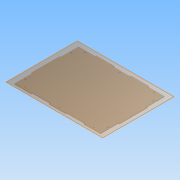
# Autodesk Inventor part: right part
Saved by Autodesk Inventor 2017 (Build 210142000, 142)
## iProperties
Part Number: right part
Material: Типовые
Document SubType Name: Modeling
Designer: Max
Mass: 338.04 g
Surface Area: 1748.93 cm^2
Volume: 338.04 cm^3
Density: 1 g/cm^3
Appearance: Поликарбонат — дымчатый
Author: Max
Autodesk Inventor part; units mm, degrees
ref_plane "YZ Plane" through (0, 0, 0) normal (1, 0, 0) x (0, 1, 0)
ref_plane "XZ Plane" through (0, 0, 0) normal (0, 1, 0) x (-1, 0, 0)
ref_plane "XY Plane" through (0, 0, 0) normal (0, 0, 1) x (1, 0, 0)
ref_plane "РабПлоскость1" through (0, 0, 0) normal (0, 0, 1) x (1, 0, 0)
sketch "Эскиз1" plane through (0, 0, 0) normal (0, 0, 1) x (1, 0, 0)
  line L0 (-1.5, 574) -> (-1.5, 579)
  line L1 (-1.5, 579) -> (-32.8, 579)
  line L2 (-32.8, 579) -> (-32.8, 583)
  line L3 (-32.8, 583) -> (-102.7, 583)
  line L4 (-102.7, 583) -> (-102.7, 579)
  line L5 (-102.7, 579) -> (-133.85, 579)
  line L6 (-133.85, 579) -> (-133.85, 574)
  line L7 (-133.85, 574) -> (-132.55, 574)
  line L8 (-132.55, 574) -> (-132.55, 571.55)
  line L9 (-132.55, 571.55) -> (-133.85, 571.55)
  line L10 (-133.85, 571.55) -> (-133.85, 570.5)
  line L11 (-133.85, 570.5) -> (-136.85, 570.5)
  line L12 (-136.85, 570.5) -> (-136.85, 571.55)
  line L13 (-136.85, 571.55) -> (-138.15, 571.55)
  line L14 (-138.15, 571.55) -> (-138.15, 574)
  line L15 (-138.15, 574) -> (-136.85, 574)
  line L16 (-136.85, 574) -> (-136.85, 579)
  line L17 (-136.85, 579) -> (-168, 579)
  line L18 (-168, 579) -> (-168, -179)
  line L19 (-168, -179) -> (168, -179)
  line L20 (168, -179) -> (168, 579)
  line L21 (168, 579) -> (136.85, 579)
  line L22 (136.85, 579) -> (136.85, 574)
  line L23 (136.85, 574) -> (138.15, 574)
  line L24 (138.15, 574) -> (138.15, 571.55)
  line L25 (138.15, 571.55) -> (136.85, 571.55)
  line L26 (136.85, 571.55) -> (136.85, 570.5)
  line L27 (136.85, 570.5) -> (133.85, 570.5)
  line L28 (133.85, 570.5) -> (133.85, 571.55)
  line L29 (133.85, 571.55) -> (132.55, 571.55)
  line L30 (132.55, 571.55) -> (132.55, 574)
  line L31 (132.55, 574) -> (133.85, 574)
  line L32 (133.85, 574) -> (133.85, 579)
  line L33 (133.85, 579) -> (102.7, 579)
  line L34 (102.7, 579) -> (102.7, 583)
  line L35 (102.7, 583) -> (32.8, 583)
  line L36 (32.8, 583) -> (32.8, 579)
  line L37 (32.8, 579) -> (1.5, 579)
  line L38 (1.5, 579) -> (1.5, 574)
  line L39 (1.5, 574) -> (2.8, 574)
  line L40 (2.8, 574) -> (2.8, 571.55)
  line L41 (2.8, 571.55) -> (1.5, 571.55)
  line L42 (1.5, 571.55) -> (1.5, 570.5)
  line L43 (1.5, 570.5) -> (-1.5, 570.5)
  line L44 (-1.5, 570.5) -> (-1.5, 571.55)
  line L45 (-1.5, 571.55) -> (-2.8, 571.55)
  line L46 (-2.8, 571.55) -> (-2.8, 574)
  line L47 (-2.8, 574) -> (-1.5, 574)
  circle A0 centre (138, 299) radius 4.75
  line L48 (-143, 100.6) -> (-143, 130)
  line L49 (-143, 130) -> (-121.6, 130)
  line L50 (-121.6, 130) -> (-121.6, 100.6)
  line L51 (-121.6, 100.6) -> (-143, 100.6)
  circle A1 centre (-156.5, 22) radius 2
  circle A2 centre (156.5, 50) radius 2
  circle A3 centre (156.5, -165) radius 2
  circle A4 centre (156.5, 132) radius 2
  circle A5 centre (-156.5, 132) radius 2
  circle A6 centre (-156.5, -165) radius 2
  circle A7 centre (158, 171) radius 5
  circle A8 centre (156, 144) radius 5
  circle A9 centre (-158, 171) radius 5
  circle A10 centre (-156, 144) radius 5
  line L52 (39.6112, -91.2079) -> (39.6112, -93.7719)
  line L53 (39.6112, -93.7719) -> (32.3927, -93.7719)
  line L54 (32.3927, -93.7719) -> (32.3927, -95.6776)
  line L55 (32.3927, -95.6776) -> (39.0914, -95.6776)
  line L56 (39.0914, -95.6776) -> (39.0914, -98.1261)
  line L57 (39.0914, -98.1261) -> (32.3927, -98.1261)
  line L58 (32.3927, -98.1261) -> (32.3927, -100.4937)
  line L59 (32.3927, -100.4937) -> (39.8191, -100.4937)
  line L60 (39.8191, -100.4937) -> (39.8191, -103.2079)
  line L61 (39.8191, -103.2079) -> (28.0847, -103.2079)
  line L62 (28.0847, -103.2079) -> (28.0847, -91.2079)
  line L63 (28.0847, -91.2079) -> (39.6112, -91.2079)
  line L64 (-2.7411, -96.3705) -> (3.9115, -96.3705)
  line L65 (3.9115, -96.3705) -> (3.9115, -101.4755)
  spline S0 degree 2 poles (3.9115, -101.4755) (2.0058, -102.6073) (-0.9278, -103.4158) (-2.949, -103.4158) knots 0 0 0 1 2 2 2
  spline S1 degree 2 poles (-2.949, -103.4158) (-5.4321, -103.4158) (-8.5505, -101.9605) (-10.2714, -99.0731) (-10.2714, -97.2021) knots 0 0 0 1 2 3 3 3
  spline S2 degree 2 poles (-10.2714, -97.2021) (-10.2714, -95.2387) (-8.3888, -92.3398) (-6.5756, -91.5775) knots 0 0 0 1 2 2 2
  spline S3 degree 2 poles (-6.5756, -91.5775) (-5.155, -91) (-2.7642, -91) knots 0 0 0 1 1 1
  spline S4 degree 2 poles (-2.7642, -91) (-0.4543, -91) (1.8325, -91.7161) (3.3455, -93.2406) (3.7267, -94.3956) knots 0 0 0 1 2 3 3 3
  line L66 (3.7267, -94.3956) -> (-0.4196, -95.0423)
  spline S5 degree 2 poles (-0.4196, -95.0423) (-0.6737, -94.3609) (-1.9095, -93.6333) (-2.8566, -93.6333) knots 0 0 0 1 2 2 2
  spline S6 degree 2 poles (-2.8566, -93.6333) (-4.2772, -93.6333) (-5.9634, -95.3311) (-5.9634, -97.1675) knots 0 0 0 1 2 2 2
  spline S7 degree 2 poles (-5.9634, -97.1675) (-5.9634, -99.1078) (-4.2541, -100.7825) (-2.7411, -100.7825) knots 0 0 0 1 2 2 2
  spline S8 degree 2 poles (-2.7411, -100.7825) (-2.0135, -100.7825) (-0.6968, -100.4244) (0.1463, -99.9856) knots 0 0 0 1 2 2 2
  line L67 (0.1463, -99.9856) -> (0.1463, -98.8653)
  line L68 (0.1463, -98.8653) -> (-2.7411, -98.8653)
  line L69 (-2.7411, -98.8653) -> (-2.7411, -96.3705)
  line L70 (-29.0279, -91.2079) -> (-29.0279, -103.2079)
  line L71 (-29.0279, -103.2079) -> (-33.3359, -103.2079)
  line L72 (-33.3359, -103.2079) -> (-33.3359, -91.2079)
  line L73 (-33.3359, -91.2079) -> (-29.0279, -91.2079)
  line L74 (-57.3128, -91.2079) -> (-57.3128, -100.2512)
  line L75 (-57.3128, -100.2512) -> (-50.591, -100.2512)
  line L76 (-50.591, -100.2512) -> (-50.591, -103.2079)
  line L77 (-50.591, -103.2079) -> (-61.6092, -103.2079)
  line L78 (-61.6092, -103.2079) -> (-61.6092, -91.2079)
  line L79 (-61.6092, -91.2079) -> (-57.3128, -91.2079)
  spline S9 degree 4 poles (-3.4576, -71.7618) (-6.8757, -71.7618) (-12.6663, -71.6289) (-17.7493, -71.4191) (-21.656, -71.1613) (-28.1265, -70.6572) (-35.7764, -69.8141) (-41.8785, -68.8111) (-43.951, -68.4597) (-46.7707, -67.9746) (-51.298, -67.0853) (-53.8623, -66.3909) (-56.6748, -65.5652) (-57.7492, -65.1092) (-58.0734, -65.1092) (-57.9243, -64.687) knots -13 -13 -13 -13 -13 -12 -11 -10 -9 -8 -7 -6 -5 -4 -3 -2 -1 -1 -1 -1 -1
  spline S10 degree 4 poles (-23.1664, -61.8343) (-26.7868, -63.6604) (-28.4505, -64.4764) (-30.3607, -65.3364) (-32.8153, -66.611) (-34.668, -67.4243) (-36.7906, -68.5248) (-40.8328, -70.2562) (-44.9088, -72.3884) (-53.4615, -75.8544) knots 1 1 1 1 1 2 3 4 5 6 7 7 7 7 7
  spline S11 degree 4 poles (-53.4615, -75.8544) (-50.4129, -73.1479) (-48.3192, -71.6289) (-46.2664, -70.4762) (-43.3421, -69.1519) (-39.3069, -67.4243) (-36.015, -66.0396) (-33.0006, -64.9417) (-31.1462, -64.2634) (-26.5466, -62.7849) (-24.2748, -62.1169) (-23.1664, -61.8343) knots 1 1 1 1 1 2 3 4 5 6 7 8 9 9 9 9 9
  spline S12 degree 4 poles (-3.4576, -71.7618) (-6.8757, -71.7618) (-12.6663, -71.6289) (-17.7493, -71.4191) (-21.656, -71.1613) (-28.1265, -70.6572) (-35.7764, -69.8141) (-41.8785, -68.8111) (-43.951, -68.4597) (-46.7707, -67.9746) (-51.298, -67.0853) (-53.8623, -66.3909) (-56.6748, -65.5652) (-57.7492, -65.1092) (-58.0734, -65.1092) (-57.9243, -64.687) knots -13 -13 -13 -13 -13 -12 -11 -10 -9 -8 -7 -6 -5 -4 -3 -2 -1 -1 -1 -1 -1
  spline S13 degree 4 poles (-3.4576, -60.3781) (-12.6161, -60.3781) (-19.753, -60.6855) (-28.028, -61.1664) (-42.3891, -62.5628) (-52.0112, -64.3309) (-62.3251, -66.0555) (-69.922, -67.9631) (-75.8067, -69.8614) (-79.183, -71.091) (-81.6689, -72.0336) (-84.2744, -72.8581) (-84.8904, -73.0917) knots -10 -10 -10 -10 -10 -9 -8 -7 -6 -5 -4 -3 -2 -1 -1 -1 -1 -1
  spline S14 degree 4 poles (-84.8904, -73.0917) (-76.086, -68.556) (-69.8517, -66.1919) (-62.9325, -64.0265) (-56.045, -62.1584) (-48.96, -60.8219) (-33.3524, -58.7017) (-24.7322, -57.7982) (-16.4787, -57.3196) (-7.3689, -57.0863) (-3.4576, -57.0863) knots -8 -8 -8 -8 -8 -7 -6 -5 -4 -3 -2 -1 -1 -1 -1 -1
  spline S15 degree 4 poles (-3.4576, -57.0863) (0.4537, -57.0863) (9.5635, -57.3196) (17.817, -57.7982) (26.4372, -58.7017) (42.0448, -60.8219) (49.1298, -62.1584) (56.0172, -64.0265) (62.9364, -66.1919) (69.1707, -68.556) (77.9751, -73.0917) knots -8 -8 -8 -8 -8 -7 -6 -5 -4 -3 -2 -1 -1 -1 -1 -1
  spline S16 degree 4 poles (77.9751, -73.0917) (77.3591, -72.8581) (74.7537, -72.0336) (72.2678, -71.091) (68.8915, -69.8614) (63.0067, -67.9631) (55.4098, -66.0555) (45.096, -64.3309) (35.4739, -62.5628) (21.1127, -61.1664) (12.8378, -60.6855) (5.7009, -60.3781) (-3.4576, -60.3781) knots -10 -10 -10 -10 -10 -9 -8 -7 -6 -5 -4 -3 -2 -1 -1 -1 -1 -1
  spline S17 degree 4 poles (51.009, -64.687) (51.1581, -65.1092) (50.8339, -65.1092) (49.7595, -65.5652) (46.947, -66.3909) (44.3828, -67.0853) (39.8554, -67.9746) (37.0358, -68.4597) (34.9633, -68.8111) (28.8611, -69.8141) (21.2113, -70.6572) (14.7407, -71.1613) (10.834, -71.4191) (5.751, -71.6289) (-0.0396, -71.7618) (-3.4576, -71.7618) knots -13 -13 -13 -13 -13 -12 -11 -10 -9 -8 -7 -6 -5 -4 -3 -2 -1 -1 -1 -1 -1
  spline S18 degree 4 poles (16.2511, -61.8343) (17.3595, -62.1169) (19.6313, -62.7849) (24.231, -64.2634) (26.0853, -64.9417) (29.0997, -66.0396) (32.3916, -67.4243) (36.4269, -69.1519) (39.3511, -70.4762) (41.404, -71.6289) (43.4976, -73.1479) (46.5463, -75.8544) knots 1 1 1 1 1 2 3 4 5 6 7 8 9 9 9 9 9
  spline S19 degree 4 poles (46.5463, -75.8544) (37.9936, -72.3884) (33.9175, -70.2562) (29.8753, -68.5248) (27.7527, -67.4243) (25.9, -66.611) (23.4454, -65.3364) (21.5352, -64.4764) (19.8716, -63.6604) (16.2511, -61.8343) knots 1 1 1 1 1 2 3 4 5 6 7 7 7 7 7
  spline S20 degree 4 poles (51.009, -64.687) (51.1581, -65.1092) (50.8339, -65.1092) (49.7595, -65.5652) (46.947, -66.3909) (44.3828, -67.0853) (39.8554, -67.9746) (37.0358, -68.4597) (34.9633, -68.8111) (28.8611, -69.8141) (21.2113, -70.6572) (14.7407, -71.1613) (10.834, -71.4191) (5.751, -71.6289) (-0.0396, -71.7618) (-3.4576, -71.7618) knots -13 -13 -13 -13 -13 -12 -11 -10 -9 -8 -7 -6 -5 -4 -3 -2 -1 -1 -1 -1 -1
  spline S21 degree 4 poles (-0.1391, -63.4469) (1.9399, -64.6408) (3.4063, -65.7041) (5.8889, -67.5053) (8.3986, -69.642) (11.5496, -72.3228) (13.0227, -73.7247) (14.943, -75.6758) (16.8187, -77.6189) (18.7978, -80.2129) (19.663, -81.5269) (20.1525, -82.3364) (20.4836, -83.1064) knots -7 -7 -7 -7 -7 -6 -5 -4 -3 -2 -1.450335 -1.166811 -1.158039 -1 -1 -1 -1 -1
  spline S22 degree 4 poles (20.4836, -83.1064) (17.2053, -79.9821) (13.5018, -76.4561) (10.178, -72.9749) (6.5451, -69.7169) (4.7293, -68.1072) (2.4529, -65.9271) (-0.1391, -63.4469) knots -5 -5 -5 -5 -5 -4 -3 -2 -1 -1 -1 -1 -1
  spline S23 degree 4 poles (51.009, -64.687) (51.1581, -65.1092) (50.8339, -65.1092) (49.7595, -65.5652) (46.947, -66.3909) (44.3828, -67.0853) (39.8554, -67.9746) (37.0358, -68.4597) (34.9633, -68.8111) (28.8611, -69.8141) (21.2113, -70.6572) (14.7407, -71.1613) (10.834, -71.4191) (5.751, -71.6289) (-0.0396, -71.7618) (-3.4576, -71.7618) knots -13 -13 -13 -13 -13 -12 -11 -10 -9 -8 -7 -6 -5 -4 -3 -2 -1 -1 -1 -1 -1
  spline S24 degree 4 poles (-3.4576, -71.7618) (-6.8757, -71.7618) (-12.6663, -71.6289) (-17.7493, -71.4191) (-21.656, -71.1613) (-28.1265, -70.6572) (-35.7764, -69.8141) (-41.8785, -68.8111) (-43.951, -68.4597) (-46.7707, -67.9746) (-51.298, -67.0853) (-53.8623, -66.3909) (-56.6748, -65.5652) (-57.7492, -65.1092) (-58.0734, -65.1092) (-57.9243, -64.687) knots -13 -13 -13 -13 -13 -12 -11 -10 -9 -8 -7 -6 -5 -4 -3 -2 -1 -1 -1 -1 -1
  spline S25 degree 4 poles (-6.7761, -63.4469) (-9.3682, -65.9271) (-11.6446, -68.1072) (-13.4603, -69.7169) (-17.0932, -72.9749) (-20.4171, -76.4561) (-24.1206, -79.9821) (-27.3989, -83.1064) knots 1 1 1 1 1 2 3 4 5 5 5 5 5
  spline S26 degree 4 poles (-27.3989, -83.1064) (-27.0678, -82.3364) (-26.5782, -81.5269) (-25.7131, -80.2129) (-23.7339, -77.6189) (-21.8583, -75.6758) (-19.9379, -73.7247) (-18.4649, -72.3228) (-15.3138, -69.642) (-12.8042, -67.5053) (-10.3215, -65.7041) (-8.8552, -64.6408) (-6.7761, -63.4469) knots 1 1 1 1 1 1.158039 1.166811 1.450335 2 3 4 5 6 7 7 7 7 7
  spline S27 degree 4 number of poles 330
  line L80 (-63.9192, -91.2079) -> (-63.9192, -93.7834)
  line L81 (-63.9192, -93.7834) -> (-70.2368, -93.7834)
  line L82 (-70.2368, -93.7834) -> (-70.2368, -95.8739)
  line L83 (-70.2368, -95.8739) -> (-64.8431, -95.8739)
  line L84 (-64.8431, -95.8739) -> (-64.8431, -98.2993)
  line L85 (-64.8431, -98.2993) -> (-70.2368, -98.2993)
  line L86 (-70.2368, -98.2993) -> (-70.2368, -103.2079)
  line L87 (-70.2368, -103.2079) -> (-74.5563, -103.2079)
  line L88 (-74.5563, -103.2079) -> (-74.5563, -91.2079)
  line L89 (-74.5563, -91.2079) -> (-63.9192, -91.2079)
  line L90 (-45.2666, -91.2079) -> (-42.4601, -95.2502)
  line L91 (-42.4601, -95.2502) -> (-39.642, -91.2079)
  line L92 (-39.642, -91.2079) -> (-34.8951, -91.2079)
  line L93 (-34.8951, -91.2079) -> (-40.3118, -98.1838)
  line L94 (-40.3118, -98.1838) -> (-40.3118, -103.2079)
  line L95 (-40.3118, -103.2079) -> (-44.6198, -103.2079)
  line L96 (-44.6198, -103.2079) -> (-44.6198, -98.1838)
  line L97 (-44.6198, -98.1838) -> (-50.0481, -91.2079)
  line L98 (-50.0481, -91.2079) -> (-45.2666, -91.2079)
  line L99 (-21.8903, -91.2079) -> (-16.6468, -97.8489)
  line L100 (-16.6468, -97.8489) -> (-16.6468, -91.2079)
  line L101 (-16.6468, -91.2079) -> (-12.5929, -91.2079)
  line L102 (-12.5929, -91.2079) -> (-12.5929, -103.2079)
  line L103 (-12.5929, -103.2079) -> (-16.6468, -103.2079)
  line L104 (-16.6468, -103.2079) -> (-21.8672, -96.6015)
  line L105 (-21.8672, -96.6015) -> (-21.8672, -103.2079)
  line L106 (-21.8672, -103.2079) -> (-25.9095, -103.2079)
  line L107 (-25.9095, -103.2079) -> (-25.9095, -91.2079)
  line L108 (-25.9095, -91.2079) -> (-21.8903, -91.2079)
  spline S28 degree 2 poles (21.0164, -91.2079) (23.026, -91.2079) (25.1858, -92.9288) (25.1858, -94.1992) knots 0 0 0 1 2 2 2
  spline S29 degree 2 poles (25.1858, -94.1992) (25.1858, -95.2618) (24.4119, -96.0241) knots 0 0 0 1 1 1
  spline S30 degree 2 poles (24.4119, -96.0241) (23.9038, -96.5322) (22.922, -96.8325) knots 0 0 0 1 1 1
  spline S31 degree 2 poles (22.922, -96.8325) (24.4119, -97.1444) (25.8325, -98.6574) (25.8325, -99.8008) knots 0 0 0 1 2 2 2
  spline S32 degree 2 poles (25.8325, -99.8008) (25.8325, -100.7247) (24.8277, -102.2146) (23.95, -102.6535) knots 0 0 0 1 2 2 2
  spline S33 degree 2 poles (23.95, -102.6535) (23.4071, -102.9192) (22.3215, -103.0462) knots 0 0 0 1 1 1
  spline S34 degree 2 poles (22.3215, -103.0462) (20.8662, -103.2079) (20.3927, -103.2079) knots 0 0 0 1 1 1
  line L109 (20.3927, -103.2079) -> (12.9663, -103.2079)
  line L110 (12.9663, -103.2079) -> (12.9663, -91.2079)
  line L111 (12.9663, -91.2079) -> (21.0164, -91.2079)
  line L112 (45.8017, -101.2214) -> (45.1203, -103.2079)
  line L113 (45.1203, -103.2079) -> (40.7199, -103.2079)
  line L114 (40.7199, -103.2079) -> (45.9519, -91.2079)
  line L115 (45.9519, -91.2079) -> (50.6641, -91.2079)
  line L116 (50.6641, -91.2079) -> (55.8845, -103.2079)
  line L117 (55.8845, -103.2079) -> (51.3802, -103.2079)
  line L118 (51.3802, -103.2079) -> (50.6872, -101.2214)
  line L119 (50.6872, -101.2214) -> (45.8017, -101.2214)
  line L120 (57.3167, -91.2079) -> (64.4889, -91.2079)
  spline S35 degree 2 poles (64.4889, -91.2079) (66.487, -91.2079) (68.589, -91.7969) (69.8826, -93.3908) (69.8826, -94.5342) knots 0 0 0 1 2 3 3 3
  spline S36 degree 2 poles (69.8826, -94.5342) (69.8826, -95.539) (68.8893, -96.9827) (68.0347, -97.4331) knots 0 0 0 1 2 2 2
  spline S37 degree 2 poles (68.0347, -97.4331) (67.4803, -97.7218) (66.5217, -97.9066) knots 0 0 0 1 1 1
  spline S38 degree 2 poles (66.5217, -97.9066) (67.2839, -98.1261) (67.642, -98.3571) knots 0 0 0 1 1 1
  spline S39 degree 2 poles (67.642, -98.3571) (67.873, -98.4957) (68.7738, -99.4658) (68.924, -99.7315) knots 0 0 0 1 2 2 2
  line L121 (68.924, -99.7315) -> (71.0144, -103.2079)
  line L122 (71.0144, -103.2079) -> (66.1521, -103.2079)
  line L123 (66.1521, -103.2079) -> (63.8537, -99.5351)
  spline S40 degree 2 poles (63.8537, -99.5351) (63.4148, -98.8306) (63.0683, -98.6112) knots 0 0 0 1 1 1
  spline S41 degree 2 poles (63.0683, -98.6112) (62.6064, -98.334) (62.0173, -98.334) knots 0 0 0 1 1 1
  line L124 (62.0173, -98.334) -> (61.6362, -98.334)
  line L125 (61.6362, -98.334) -> (61.6362, -103.2079)
  line L126 (61.6362, -103.2079) -> (57.3167, -103.2079)
  line L127 (57.3167, -103.2079) -> (57.3167, -91.2079)
  line L128 (-1.5, 324) -> (-1.5, 329)
  line L129 (-1.5, 329) -> (-32.8, 329)
  line L130 (-32.8, 329) -> (-32.8, 333)
  line L131 (-32.8, 333) -> (-102.7, 333)
  line L132 (-102.7, 333) -> (-102.7, 329)
  line L133 (-102.7, 329) -> (-133.85, 329)
  line L134 (-133.85, 329) -> (-133.85, 324)
  line L135 (-133.85, 324) -> (-132.55, 324)
  line L136 (-132.55, 324) -> (-132.55, 321.55)
  line L137 (-132.55, 321.55) -> (-133.85, 321.55)
  line L138 (-133.85, 321.55) -> (-133.85, 320.5)
  line L139 (-133.85, 320.5) -> (-136.85, 320.5)
  line L140 (-136.85, 320.5) -> (-136.85, 321.55)
  line L141 (-136.85, 321.55) -> (-138.15, 321.55)
  line L142 (-138.15, 321.55) -> (-138.15, 324)
  line L143 (-138.15, 324) -> (-136.85, 324)
  line L144 (-136.85, 324) -> (-136.85, 329)
  line L145 (-136.85, 329) -> (-168, 329)
  line L146 (-168, 329) -> (-168, -179)
  line L147 (-168, -179) -> (168, -179)
  line L148 (168, -179) -> (168, 329)
  line L149 (168, 329) -> (136.85, 329)
  line L150 (136.85, 329) -> (136.85, 324)
  line L151 (136.85, 324) -> (138.15, 324)
  line L152 (138.15, 324) -> (138.15, 321.55)
  line L153 (138.15, 321.55) -> (136.85, 321.55)
  line L154 (136.85, 321.55) -> (136.85, 320.5)
  line L155 (136.85, 320.5) -> (133.85, 320.5)
  line L156 (133.85, 320.5) -> (133.85, 321.55)
  line L157 (133.85, 321.55) -> (132.55, 321.55)
  line L158 (132.55, 321.55) -> (132.55, 324)
  line L159 (132.55, 324) -> (133.85, 324)
  line L160 (133.85, 324) -> (133.85, 329)
  line L161 (133.85, 329) -> (102.7, 329)
  line L162 (102.7, 329) -> (102.7, 333) construction
  line L163 (102.7, 333) -> (32.8, 333)
  line L164 (32.8, 333) -> (32.8, 329)
  line L165 (32.8, 329) -> (1.5, 329)
  line L166 (1.5, 329) -> (1.5, 324)
  line L167 (1.5, 324) -> (2.8, 324)
  line L168 (2.8, 324) -> (2.8, 321.55)
  line L169 (2.8, 321.55) -> (1.5, 321.55)
  line L170 (1.5, 321.55) -> (1.5, 320.5)
  line L171 (1.5, 320.5) -> (-1.5, 320.5)
  line L172 (-1.5, 320.5) -> (-1.5, 321.55)
  line L173 (-1.5, 321.55) -> (-2.8, 321.55)
  line L174 (-2.8, 321.55) -> (-2.8, 324)
  line L175 (-2.8, 324) -> (-1.5, 324)
  circle A11 centre (138, 299) radius 4.75
  line L176 (-143, 100.6) -> (-143, 130)
  line L177 (-143, 130) -> (-121.6, 130)
  line L178 (-121.6, 130) -> (-121.6, 100.6)
  line L179 (-121.6, 100.6) -> (-143, 100.6)
  circle A12 centre (-156.5, 22) radius 2
  circle A13 centre (156.5, 50) radius 2
  circle A14 centre (156.5, -165) radius 2
  circle A15 centre (156.5, 132) radius 2
  circle A16 centre (-156.5, 132) radius 2
  circle A17 centre (-156.5, -165) radius 2
  circle A18 centre (158, 171) radius 5
  circle A19 centre (156, 144) radius 5
  circle A20 centre (-158, 171) radius 5
  circle A21 centre (-156, 144) radius 5
  line L180 (39.6112, -91.2079) -> (39.6112, -93.7719)
  line L181 (39.6112, -93.7719) -> (32.3927, -93.7719)
  line L182 (32.3927, -93.7719) -> (32.3927, -95.6776)
  line L183 (32.3927, -95.6776) -> (39.0914, -95.6776)
  line L184 (39.0914, -95.6776) -> (39.0914, -98.1261)
  line L185 (39.0914, -98.1261) -> (32.3927, -98.1261)
  line L186 (32.3927, -98.1261) -> (32.3927, -100.4937)
  line L187 (32.3927, -100.4937) -> (39.8191, -100.4937)
  line L188 (39.8191, -100.4937) -> (39.8191, -103.2079)
  line L189 (39.8191, -103.2079) -> (28.0847, -103.2079)
  line L190 (28.0847, -103.2079) -> (28.0847, -91.2079)
  line L191 (28.0847, -91.2079) -> (39.6112, -91.2079)
  line L192 (-2.7411, -96.3705) -> (3.9115, -96.3705)
  line L193 (3.9115, -96.3705) -> (3.9115, -101.4755)
  spline S42 degree 2 poles (3.9115, -101.4755) (2.0058, -102.6073) (-0.9278, -103.4158) (-2.949, -103.4158) knots 0 0 0 1 2 2 2
  spline S43 degree 2 poles (-2.949, -103.4158) (-5.4321, -103.4158) (-8.5505, -101.9605) (-10.2714, -99.0731) (-10.2714, -97.2021) knots 0 0 0 1 2 3 3 3
  spline S44 degree 2 poles (-10.2714, -97.2021) (-10.2714, -95.2387) (-8.3888, -92.3398) (-6.5756, -91.5775) knots 0 0 0 1 2 2 2
  spline S45 degree 2 poles (-6.5756, -91.5775) (-5.155, -91) (-2.7642, -91) knots 0 0 0 1 1 1
  spline S46 degree 2 poles (-2.7642, -91) (-0.4543, -91) (1.8325, -91.7161) (3.3455, -93.2406) (3.7267, -94.3956) knots 0 0 0 1 2 3 3 3
  line L194 (3.7267, -94.3956) -> (-0.4196, -95.0423)
  spline S47 degree 2 poles (-0.4196, -95.0423) (-0.6737, -94.3609) (-1.9095, -93.6333) (-2.8566, -93.6333) knots 0 0 0 1 2 2 2
  spline S48 degree 2 poles (-2.8566, -93.6333) (-4.2772, -93.6333) (-5.9634, -95.3311) (-5.9634, -97.1675) knots 0 0 0 1 2 2 2
  spline S49 degree 2 poles (-5.9634, -97.1675) (-5.9634, -99.1078) (-4.2541, -100.7825) (-2.7411, -100.7825) knots 0 0 0 1 2 2 2
  spline S50 degree 2 poles (-2.7411, -100.7825) (-2.0135, -100.7825) (-0.6968, -100.4244) (0.1463, -99.9856) knots 0 0 0 1 2 2 2
  line L195 (0.1463, -99.9856) -> (0.1463, -98.8653)
  line L196 (0.1463, -98.8653) -> (-2.7411, -98.8653)
  line L197 (-2.7411, -98.8653) -> (-2.7411, -96.3705)
  line L198 (-29.0279, -91.2079) -> (-29.0279, -103.2079)
  line L199 (-29.0279, -103.2079) -> (-33.3359, -103.2079)
  line L200 (-33.3359, -103.2079) -> (-33.3359, -91.2079)
  line L201 (-33.3359, -91.2079) -> (-29.0279, -91.2079)
  line L202 (-57.3128, -91.2079) -> (-57.3128, -100.2512)
  line L203 (-57.3128, -100.2512) -> (-50.591, -100.2512)
  line L204 (-50.591, -100.2512) -> (-50.591, -103.2079)
  line L205 (-50.591, -103.2079) -> (-61.6092, -103.2079)
  line L206 (-61.6092, -103.2079) -> (-61.6092, -91.2079)
  line L207 (-61.6092, -91.2079) -> (-57.3128, -91.2079)
  spline S51 degree 4 poles (-3.4576, -71.7618) (-6.8757, -71.7618) (-12.6663, -71.6289) (-17.7493, -71.4191) (-21.656, -71.1613) (-28.1265, -70.6572) (-35.7764, -69.8141) (-41.8785, -68.8111) (-43.951, -68.4597) (-46.7707, -67.9746) (-51.298, -67.0853) (-53.8623, -66.3909) (-56.6748, -65.5652) (-57.7492, -65.1092) (-58.0734, -65.1092) (-57.9243, -64.687) knots -13 -13 -13 -13 -13 -12 -11 -10 -9 -8 -7 -6 -5 -4 -3 -2 -1 -1 -1 -1 -1
  spline S52 degree 4 poles (-23.1664, -61.8343) (-26.7868, -63.6604) (-28.4505, -64.4764) (-30.3607, -65.3364) (-32.8153, -66.611) (-34.668, -67.4243) (-36.7906, -68.5248) (-40.8328, -70.2562) (-44.9088, -72.3884) (-53.4615, -75.8544) knots 1 1 1 1 1 2 3 4 5 6 7 7 7 7 7
  spline S53 degree 4 poles (-53.4615, -75.8544) (-50.4129, -73.1479) (-48.3192, -71.6289) (-46.2664, -70.4762) (-43.3421, -69.1519) (-39.3069, -67.4243) (-36.015, -66.0396) (-33.0006, -64.9417) (-31.1462, -64.2634) (-26.5466, -62.7849) (-24.2748, -62.1169) (-23.1664, -61.8343) knots 1 1 1 1 1 2 3 4 5 6 7 8 9 9 9 9 9
  spline S54 degree 4 poles (-3.4576, -71.7618) (-6.8757, -71.7618) (-12.6663, -71.6289) (-17.7493, -71.4191) (-21.656, -71.1613) (-28.1265, -70.6572) (-35.7764, -69.8141) (-41.8785, -68.8111) (-43.951, -68.4597) (-46.7707, -67.9746) (-51.298, -67.0853) (-53.8623, -66.3909) (-56.6748, -65.5652) (-57.7492, -65.1092) (-58.0734, -65.1092) (-57.9243, -64.687) knots -13 -13 -13 -13 -13 -12 -11 -10 -9 -8 -7 -6 -5 -4 -3 -2 -1 -1 -1 -1 -1
  spline S55 degree 4 poles (-3.4576, -60.3781) (-12.6161, -60.3781) (-19.753, -60.6855) (-28.028, -61.1664) (-42.3891, -62.5628) (-52.0112, -64.3309) (-62.3251, -66.0555) (-69.922, -67.9631) (-75.8067, -69.8614) (-79.183, -71.091) (-81.6689, -72.0336) (-84.2744, -72.8581) (-84.8904, -73.0917) knots -10 -10 -10 -10 -10 -9 -8 -7 -6 -5 -4 -3 -2 -1 -1 -1 -1 -1
  spline S56 degree 4 poles (-84.8904, -73.0917) (-76.086, -68.556) (-69.8517, -66.1919) (-62.9325, -64.0265) (-56.045, -62.1584) (-48.96, -60.8219) (-33.3524, -58.7017) (-24.7322, -57.7982) (-16.4787, -57.3196) (-7.3689, -57.0863) (-3.4576, -57.0863) knots -8 -8 -8 -8 -8 -7 -6 -5 -4 -3 -2 -1 -1 -1 -1 -1
  spline S57 degree 4 poles (-3.4576, -57.0863) (0.4537, -57.0863) (9.5635, -57.3196) (17.817, -57.7982) (26.4372, -58.7017) (42.0448, -60.8219) (49.1298, -62.1584) (56.0172, -64.0265) (62.9364, -66.1919) (69.1707, -68.556) (77.9751, -73.0917) knots -8 -8 -8 -8 -8 -7 -6 -5 -4 -3 -2 -1 -1 -1 -1 -1
  spline S58 degree 4 poles (77.9751, -73.0917) (77.3591, -72.8581) (74.7537, -72.0336) (72.2678, -71.091) (68.8915, -69.8614) (63.0067, -67.9631) (55.4098, -66.0555) (45.096, -64.3309) (35.4739, -62.5628) (21.1127, -61.1664) (12.8378, -60.6855) (5.7009, -60.3781) (-3.4576, -60.3781) knots -10 -10 -10 -10 -10 -9 -8 -7 -6 -5 -4 -3 -2 -1 -1 -1 -1 -1
  spline S59 degree 4 poles (51.009, -64.687) (51.1581, -65.1092) (50.8339, -65.1092) (49.7595, -65.5652) (46.947, -66.3909) (44.3828, -67.0853) (39.8554, -67.9746) (37.0358, -68.4597) (34.9633, -68.8111) (28.8611, -69.8141) (21.2113, -70.6572) (14.7407, -71.1613) (10.834, -71.4191) (5.751, -71.6289) (-0.0396, -71.7618) (-3.4576, -71.7618) knots -13 -13 -13 -13 -13 -12 -11 -10 -9 -8 -7 -6 -5 -4 -3 -2 -1 -1 -1 -1 -1
  spline S60 degree 4 poles (16.2511, -61.8343) (17.3595, -62.1169) (19.6313, -62.7849) (24.231, -64.2634) (26.0853, -64.9417) (29.0997, -66.0396) (32.3916, -67.4243) (36.4269, -69.1519) (39.3511, -70.4762) (41.404, -71.6289) (43.4976, -73.1479) (46.5463, -75.8544) knots 1 1 1 1 1 2 3 4 5 6 7 8 9 9 9 9 9
  spline S61 degree 4 poles (46.5463, -75.8544) (37.9936, -72.3884) (33.9175, -70.2562) (29.8753, -68.5248) (27.7527, -67.4243) (25.9, -66.611) (23.4454, -65.3364) (21.5352, -64.4764) (19.8716, -63.6604) (16.2511, -61.8343) knots 1 1 1 1 1 2 3 4 5 6 7 7 7 7 7
  spline S62 degree 4 poles (51.009, -64.687) (51.1581, -65.1092) (50.8339, -65.1092) (49.7595, -65.5652) (46.947, -66.3909) (44.3828, -67.0853) (39.8554, -67.9746) (37.0358, -68.4597) (34.9633, -68.8111) (28.8611, -69.8141) (21.2113, -70.6572) (14.7407, -71.1613) (10.834, -71.4191) (5.751, -71.6289) (-0.0396, -71.7618) (-3.4576, -71.7618) knots -13 -13 -13 -13 -13 -12 -11 -10 -9 -8 -7 -6 -5 -4 -3 -2 -1 -1 -1 -1 -1
  spline S63 degree 4 poles (-0.1391, -63.4469) (1.9399, -64.6408) (3.4063, -65.7041) (5.8889, -67.5053) (8.3986, -69.642) (11.5496, -72.3228) (13.0227, -73.7247) (14.943, -75.6758) (16.8187, -77.6189) (18.7978, -80.2129) (19.663, -81.5269) (20.1525, -82.3364) (20.4836, -83.1064) knots -7 -7 -7 -7 -7 -6 -5 -4 -3 -2 -1.450335 -1.166811 -1.158039 -1 -1 -1 -1 -1
  spline S64 degree 4 poles (20.4836, -83.1064) (17.2053, -79.9821) (13.5018, -76.4561) (10.178, -72.9749) (6.5451, -69.7169) (4.7293, -68.1072) (2.4529, -65.9271) (-0.1391, -63.4469) knots -5 -5 -5 -5 -5 -4 -3 -2 -1 -1 -1 -1 -1
  spline S65 degree 4 poles (51.009, -64.687) (51.1581, -65.1092) (50.8339, -65.1092) (49.7595, -65.5652) (46.947, -66.3909) (44.3828, -67.0853) (39.8554, -67.9746) (37.0358, -68.4597) (34.9633, -68.8111) (28.8611, -69.8141) (21.2113, -70.6572) (14.7407, -71.1613) (10.834, -71.4191) (5.751, -71.6289) (-0.0396, -71.7618) (-3.4576, -71.7618) knots -13 -13 -13 -13 -13 -12 -11 -10 -9 -8 -7 -6 -5 -4 -3 -2 -1 -1 -1 -1 -1
  spline S66 degree 4 poles (-3.4576, -71.7618) (-6.8757, -71.7618) (-12.6663, -71.6289) (-17.7493, -71.4191) (-21.656, -71.1613) (-28.1265, -70.6572) (-35.7764, -69.8141) (-41.8785, -68.8111) (-43.951, -68.4597) (-46.7707, -67.9746) (-51.298, -67.0853) (-53.8623, -66.3909) (-56.6748, -65.5652) (-57.7492, -65.1092) (-58.0734, -65.1092) (-57.9243, -64.687) knots -13 -13 -13 -13 -13 -12 -11 -10 -9 -8 -7 -6 -5 -4 -3 -2 -1 -1 -1 -1 -1
  spline S67 degree 4 poles (-6.7761, -63.4469) (-9.3682, -65.9271) (-11.6446, -68.1072) (-13.4603, -69.7169) (-17.0932, -72.9749) (-20.4171, -76.4561) (-24.1206, -79.9821) (-27.3989, -83.1064) knots 1 1 1 1 1 2 3 4 5 5 5 5 5
  spline S68 degree 4 poles (-27.3989, -83.1064) (-27.0678, -82.3364) (-26.5782, -81.5269) (-25.7131, -80.2129) (-23.7339, -77.6189) (-21.8583, -75.6758) (-19.9379, -73.7247) (-18.4649, -72.3228) (-15.3138, -69.642) (-12.8042, -67.5053) (-10.3215, -65.7041) (-8.8552, -64.6408) (-6.7761, -63.4469) knots 1 1 1 1 1 1.158039 1.166811 1.450335 2 3 4 5 6 7 7 7 7 7
  spline S69 degree 4 number of poles 330
  line L208 (-63.9192, -91.2079) -> (-63.9192, -93.7834)
  line L209 (-63.9192, -93.7834) -> (-70.2368, -93.7834)
  line L210 (-70.2368, -93.7834) -> (-70.2368, -95.8739)
  line L211 (-70.2368, -95.8739) -> (-64.8431, -95.8739)
  line L212 (-64.8431, -95.8739) -> (-64.8431, -98.2993)
  line L213 (-64.8431, -98.2993) -> (-70.2368, -98.2993)
  line L214 (-70.2368, -98.2993) -> (-70.2368, -103.2079)
  line L215 (-70.2368, -103.2079) -> (-74.5563, -103.2079)
  line L216 (-74.5563, -103.2079) -> (-74.5563, -91.2079)
  line L217 (-74.5563, -91.2079) -> (-63.9192, -91.2079)
  line L218 (-45.2666, -91.2079) -> (-42.4601, -95.2502)
  line L219 (-42.4601, -95.2502) -> (-39.642, -91.2079)
  line L220 (-39.642, -91.2079) -> (-34.8951, -91.2079)
  line L221 (-34.8951, -91.2079) -> (-40.3118, -98.1838)
  line L222 (-40.3118, -98.1838) -> (-40.3118, -103.2079)
  line L223 (-40.3118, -103.2079) -> (-44.6198, -103.2079)
  line L224 (-44.6198, -103.2079) -> (-44.6198, -98.1838)
  line L225 (-44.6198, -98.1838) -> (-50.0481, -91.2079)
  line L226 (-50.0481, -91.2079) -> (-45.2666, -91.2079)
  line L227 (-21.8903, -91.2079) -> (-16.6468, -97.8489)
  line L228 (-16.6468, -97.8489) -> (-16.6468, -91.2079)
  line L229 (-16.6468, -91.2079) -> (-12.5929, -91.2079)
  line L230 (-12.5929, -91.2079) -> (-12.5929, -103.2079)
  line L231 (-12.5929, -103.2079) -> (-16.6468, -103.2079)
  line L232 (-16.6468, -103.2079) -> (-21.8672, -96.6015)
  line L233 (-21.8672, -96.6015) -> (-21.8672, -103.2079)
  line L234 (-21.8672, -103.2079) -> (-25.9095, -103.2079)
  line L235 (-25.9095, -103.2079) -> (-25.9095, -91.2079)
  line L236 (-25.9095, -91.2079) -> (-21.8903, -91.2079)
  spline S70 degree 2 poles (21.0164, -91.2079) (23.026, -91.2079) (25.1858, -92.9288) (25.1858, -94.1992) knots 0 0 0 1 2 2 2
  spline S71 degree 2 poles (25.1858, -94.1992) (25.1858, -95.2618) (24.4119, -96.0241) knots 0 0 0 1 1 1
  spline S72 degree 2 poles (24.4119, -96.0241) (23.9038, -96.5322) (22.922, -96.8325) knots 0 0 0 1 1 1
  spline S73 degree 2 poles (22.922, -96.8325) (24.4119, -97.1444) (25.8325, -98.6574) (25.8325, -99.8008) knots 0 0 0 1 2 2 2
  spline S74 degree 2 poles (25.8325, -99.8008) (25.8325, -100.7247) (24.8277, -102.2146) (23.95, -102.6535) knots 0 0 0 1 2 2 2
  spline S75 degree 2 poles (23.95, -102.6535) (23.4071, -102.9192) (22.3215, -103.0462) knots 0 0 0 1 1 1
  spline S76 degree 2 poles (22.3215, -103.0462) (20.8662, -103.2079) (20.3927, -103.2079) knots 0 0 0 1 1 1
  line L237 (20.3927, -103.2079) -> (12.9663, -103.2079)
  line L238 (12.9663, -103.2079) -> (12.9663, -91.2079)
  line L239 (12.9663, -91.2079) -> (21.0164, -91.2079)
  line L240 (45.8017, -101.2214) -> (45.1203, -103.2079)
  line L241 (45.1203, -103.2079) -> (40.7199, -103.2079)
  line L242 (40.7199, -103.2079) -> (45.9519, -91.2079)
  line L243 (45.9519, -91.2079) -> (50.6641, -91.2079)
  line L244 (50.6641, -91.2079) -> (55.8845, -103.2079)
  line L245 (55.8845, -103.2079) -> (51.3802, -103.2079)
  line L246 (51.3802, -103.2079) -> (50.6872, -101.2214)
  line L247 (50.6872, -101.2214) -> (45.8017, -101.2214)
  line L248 (57.3167, -91.2079) -> (64.4889, -91.2079)
  spline S77 degree 2 poles (64.4889, -91.2079) (66.487, -91.2079) (68.589, -91.7969) (69.8826, -93.3908) (69.8826, -94.5342) knots 0 0 0 1 2 3 3 3
  spline S78 degree 2 poles (69.8826, -94.5342) (69.8826, -95.539) (68.8893, -96.9827) (68.0347, -97.4331) knots 0 0 0 1 2 2 2
  spline S79 degree 2 poles (68.0347, -97.4331) (67.4803, -97.7218) (66.5217, -97.9066) knots 0 0 0 1 1 1
  spline S80 degree 2 poles (66.5217, -97.9066) (67.2839, -98.1261) (67.642, -98.3571) knots 0 0 0 1 1 1
  spline S81 degree 2 poles (67.642, -98.3571) (67.873, -98.4957) (68.7738, -99.4658) (68.924, -99.7315) knots 0 0 0 1 2 2 2
  line L249 (68.924, -99.7315) -> (71.0144, -103.2079)
  line L250 (71.0144, -103.2079) -> (66.1521, -103.2079)
  line L251 (66.1521, -103.2079) -> (63.8537, -99.5351)
  spline S82 degree 2 poles (63.8537, -99.5351) (63.4148, -98.8306) (63.0683, -98.6112) knots 0 0 0 1 1 1
  spline S83 degree 2 poles (63.0683, -98.6112) (62.6064, -98.334) (62.0173, -98.334) knots 0 0 0 1 1 1
  line L252 (62.0173, -98.334) -> (61.6362, -98.334)
  line L253 (61.6362, -98.334) -> (61.6362, -103.2079)
  line L254 (61.6362, -103.2079) -> (57.3167, -103.2079)
  line L255 (57.3167, -103.2079) -> (57.3167, -91.2079)
  line L256 (-163, 336) -> (158, 336) construction
  line L257 (-136.85, 329) -> (-133.85, 329)
  line L258 (-1.5, 329) -> (1.5, 329)
  line L259 (133.85, 329) -> (136.85, 329)
  line L260 (-135.35, 329) -> (-135.35, 336) construction
  line L261 (0, 329) -> (0, 336) construction
  line L262 (135.35, 329) -> (135.35, 336) construction
  circle A22 centre (135.35, 336) radius 1.55
  circle A23 centre (0, 336) radius 1.55
  circle A24 centre (-135.35, 336) radius 1.55
  line L263 (-102.7, 333) -> (-102.8, 333)
  line L264 (-102.8, 333) -> (-102.8, 329)
  line L265 (-102.8, 329) -> (-102.7, 329)
  line L266 (-102.7, 329) -> (-102.7, 333)
  line L267 (-32.8, 333) -> (-32.7, 333)
  line L268 (-32.7, 333) -> (-32.7, 329)
  line L269 (-32.7, 329) -> (-32.8, 329)
  line L270 (-32.8, 329) -> (-32.8, 333)
  line L271 (32.8, 333) -> (32.7, 333)
  line L272 (32.7, 333) -> (32.7, 329)
  line L273 (32.7, 329) -> (32.8, 329)
  line L274 (32.8, 329) -> (32.8, 333)
  line L275 (102.7, 333) -> (102.8, 333)
  line L276 (102.8, 333) -> (102.8, 329)
  line L277 (102.8, 329) -> (102.7, 329)
  line L278 (102.7, 329) -> (102.7, 333)
  point P0 (0, 0)
  point P1 (-32.2045, 31.6908)
  dimension "d0" = 4
  dimension "d1" = 5
  dimension "d2" = 2.45
  dimension "d3" = 1.05
  dimension "d4" = 250
  dimension "d5" = 7
  dimension "d6" = 3.1
  dimension "d7" = 3.1
  dimension "d8" = 3.1
  dimension "d9" = 0.1
  dimension "d10" = 0.1
  dimension "d11" = 0.1
  dimension "d12" = 0.1
  constraints: 136 end point, 18 collinear, 10 equal length, 7 perpendicular, 6 horizontal, 6 point on line, 3 centre point, 3 coincident, 3 midpoint
  measures "d0" distance between parallel lines of L1 L3
  measures "d1" distance between parallel lines of L39 L37
  measures "d2" distance between parallel lines of L41 L39
  measures "d3" distance between parallel lines of L43 L41
  measures "d4" distance between parallel lines of L131 L3
  measures "d5" distance between parallel lines of L161 L256
  measures "d6" diameter of A22
  measures "d7" diameter of A23
  measures "d8" diameter of A24
  measures "d9" distance between parallel lines of L132 L264
  measures "d10" distance between parallel lines of L130 L268
  measures "d11" distance between parallel lines of L274 L272
  measures "d12" distance between parallel lines of L276 L162
extrude "Выдавливание1" add sketch "Эскиз1" against normal blind 4 contours L47 L46 L45 L44 L43 L42 L41 L40 L39 L38 L37 L36 L35 L34 L33 L32 L31 L30 L29 L28 L27 L26 L25 L24 L23 L22 L21 L20 L149 L259 L161 L276 L275 L163 L271 L272 L165 L258 L129 L268 L267 L131 L263 L264 L133 L257 L145 L18 L17 L16 L15 L14 L13 L12 L11 L10 L9 L8 L7 L6 L5 L4 L3 L2 L1 L0
sketch "Эскиз4" plane through (0, 0, 0) normal (0, 0, 1) x (1, 0, 0)
  circle A0 centre (-32, 364) radius 4
  circle A1 centre (118, 364) radius 4
  line L0 (43, 461.2299) -> (43, 364)
  line L1 (-32, 364) -> (118, 364) construction
  line L2 (-32.7, 329) -> (32.7, 329) construction
  line L3 (168, 329) -> (168, 579) projected
  point P0 (0, 0)
  dimension "d15" = 8
  dimension "d16" = 8
  dimension "d17" = 150
  dimension "d18" = 35
  dimension "d21" = 125
  constraints: 4 end point, 2 centre point, 1 horizontal, 1 midpoint, 1 symmetric about line, 1 vertical
  measures "d15" diameter of A0
  measures "d16" diameter of A1
  measures "d17" distance of L1.end L1.start
  measures "d18" distance from line of L1.start L2
  measures "d21" distance from line of L3 L0.end
extrude "Выдавливание2" cut sketch "Эскиз4" against normal blind 4
sketch "Эскиз5" plane through (0, 0, 0) normal (0, 0, 1) x (1, 0, 0)
  circle A0 centre (-32, 364) radius 4 projected
  circle A1 centre (118, 364) radius 4 projected
  circle A2 centre (-135.35, 336) radius 1.55 projected
  circle A3 centre (0, 336) radius 1.55 projected
  circle A4 centre (135.35, 336) radius 1.55 projected
  line L0 (-102.8, 329) -> (-102.8, 333) projected
  line L1 (-102.8, 333) -> (-32.7, 333) projected
  line L2 (-32.7, 333) -> (-32.7, 329) projected
  line L3 (-32.7, 329) -> (32.7, 329) projected
  line L4 (32.7, 329) -> (32.7, 333) projected
  line L5 (32.7, 333) -> (102.8, 333) projected
  line L6 (102.8, 333) -> (102.8, 329) projected
  line L7 (102.8, 329) -> (168, 329) projected
  line L8 (168, 329) -> (168, 579) projected
  line L9 (168, 579) -> (136.85, 579) projected
  line L10 (136.85, 579) -> (136.85, 574) projected
  line L11 (136.85, 574) -> (138.15, 574) projected
  line L12 (138.15, 574) -> (138.15, 571.55) projected
  line L13 (138.15, 571.55) -> (136.85, 571.55) projected
  line L14 (136.85, 571.55) -> (136.85, 570.5) projected
  line L15 (136.85, 570.5) -> (133.85, 570.5) projected
  line L16 (133.85, 570.5) -> (133.85, 571.55) projected
  line L17 (133.85, 571.55) -> (132.55, 571.55) projected
  line L18 (132.55, 571.55) -> (132.55, 574) projected
  line L19 (132.55, 574) -> (133.85, 574) projected
  line L20 (133.85, 574) -> (133.85, 579) projected
  line L21 (133.85, 579) -> (102.7, 579) projected
  line L22 (102.7, 579) -> (102.7, 583) projected
  line L23 (102.7, 583) -> (32.8, 583) projected
  line L24 (32.8, 583) -> (32.8, 579) projected
  line L25 (32.8, 579) -> (1.5, 579) projected
  line L26 (1.5, 579) -> (1.5, 574) projected
  line L27 (1.5, 574) -> (2.8, 574) projected
  line L28 (2.8, 574) -> (2.8, 571.55) projected
  line L29 (2.8, 571.55) -> (1.5, 571.55) projected
  line L30 (1.5, 571.55) -> (1.5, 570.5) projected
  line L31 (1.5, 570.5) -> (-1.5, 570.5) projected
  line L32 (-1.5, 570.5) -> (-1.5, 571.55) projected
  line L33 (-1.5, 571.55) -> (-2.8, 571.55) projected
  line L34 (-2.8, 571.55) -> (-2.8, 574) projected
  line L35 (-2.8, 574) -> (-1.5, 574) projected
  line L36 (-1.5, 574) -> (-1.5, 579) projected
  line L37 (-1.5, 579) -> (-32.8, 579) projected
  line L38 (-32.8, 579) -> (-32.8, 583) projected
  line L39 (-32.8, 583) -> (-102.7, 583) projected
  line L40 (-102.7, 583) -> (-102.7, 579) projected
  line L41 (-102.7, 579) -> (-133.85, 579) projected
  line L42 (-133.85, 579) -> (-133.85, 574) projected
  line L43 (-133.85, 574) -> (-132.55, 574) projected
  line L44 (-132.55, 574) -> (-132.55, 571.55) projected
  line L45 (-132.55, 571.55) -> (-133.85, 571.55) projected
  line L46 (-133.85, 571.55) -> (-133.85, 570.5) projected
  line L47 (-133.85, 570.5) -> (-136.85, 570.5) projected
  line L48 (-136.85, 570.5) -> (-136.85, 571.55) projected
  line L49 (-136.85, 571.55) -> (-138.15, 571.55) projected
  line L50 (-138.15, 571.55) -> (-138.15, 574) projected
  line L51 (-138.15, 574) -> (-136.85, 574) projected
  line L52 (-136.85, 574) -> (-136.85, 579) projected
  line L53 (-136.85, 579) -> (-168, 579) projected
  line L54 (-168, 579) -> (-168, 329) projected
  line L55 (-168, 329) -> (-102.8, 329) projected
  line L56 (-168, 329) -> (-168, 579) projected
  line L57 (-168, 509) -> (-172, 509)
  line L58 (-172, 509) -> (-172, 399)
  line L59 (-172, 399) -> (-168, 399)
  line L60 (-168, 399) -> (-168, 509)
  line L61 (168, 579) -> (168, 329) projected
  line L62 (168, 509) -> (172, 509)
  line L63 (172, 509) -> (172, 399)
  line L64 (172, 399) -> (168, 399)
  line L65 (168, 399) -> (168, 509)
  line L66 (-136.85, 579) -> (-168, 579) projected
  line L67 (-168, 509) -> (-168, 579)
  line L68 (-168, 544) -> (-154, 544) construction
  line L69 (-168, 545.5) -> (-163, 545.5)
  line L70 (-163, 545.5) -> (-163, 546.8)
  line L71 (-163, 546.8) -> (-160.55, 546.8)
  line L72 (-160.55, 546.8) -> (-160.55, 545.5)
  line L73 (-160.55, 545.5) -> (-159.5, 545.5)
  line L74 (-159.5, 545.5) -> (-159.5, 542.5)
  line L75 (-159.5, 542.5) -> (-160.55, 542.5)
  line L76 (-160.55, 542.5) -> (-160.55, 541.2)
  line L77 (-160.55, 541.2) -> (-163, 541.2)
  line L78 (-163, 541.2) -> (-163, 542.5)
  line L79 (-168, 542.5) -> (-163, 542.5)
  line L80 (-168, 399) -> (-168, 329)
  line L81 (-168, 364) -> (-144, 364) construction
  line L82 (-168, 184) -> (-144, 184) construction
  line L83 (-159.5, 362.5) -> (-160.55, 362.5)
  line L84 (-168, 362.5) -> (-163, 362.5)
  line L85 (-160.55, 362.5) -> (-160.55, 361.2)
  line L86 (-160.55, 361.2) -> (-163, 361.2)
  line L87 (-163, 361.2) -> (-163, 362.5)
  line L88 (-159.5, 365.5) -> (-159.5, 362.5)
  line L89 (-168, 364) -> (-154, 364) construction
  line L90 (-168, 365.5) -> (-163, 365.5)
  line L91 (-160.55, 365.5) -> (-159.5, 365.5)
  line L92 (-163, 365.5) -> (-163, 366.8)
  line L93 (-160.55, 366.8) -> (-160.55, 365.5)
  line L94 (-163, 366.8) -> (-160.55, 366.8)
  line L95 (-168, 365.5) -> (-168, 362.5)
  line L96 (32.7, 329) -> (-32.7, 329) projected
  line L97 (0, 329) -> (0, 384)
  line L98 (168, 544) -> (154, 544) construction
  line L99 (168, 545.5) -> (163, 545.5)
  line L100 (163, 545.5) -> (163, 546.8)
  line L101 (163, 546.8) -> (160.55, 546.8)
  line L102 (160.55, 546.8) -> (160.55, 545.5)
  line L103 (160.55, 545.5) -> (159.5, 545.5)
  line L104 (159.5, 545.5) -> (159.5, 542.5)
  line L105 (159.5, 542.5) -> (160.55, 542.5)
  line L106 (160.55, 542.5) -> (160.55, 541.2)
  line L107 (160.55, 541.2) -> (163, 541.2)
  line L108 (163, 541.2) -> (163, 542.5)
  line L109 (168, 542.5) -> (163, 542.5)
  line L110 (159.5, 362.5) -> (160.55, 362.5)
  line L111 (168, 362.5) -> (163, 362.5)
  line L112 (160.55, 362.5) -> (160.55, 361.2)
  line L113 (160.55, 361.2) -> (163, 361.2)
  line L114 (163, 361.2) -> (163, 362.5)
  line L115 (159.5, 365.5) -> (159.5, 362.5)
  line L116 (168, 364) -> (154, 364) construction
  line L117 (168, 365.5) -> (163, 365.5)
  line L118 (160.55, 365.5) -> (159.5, 365.5)
  line L119 (163, 365.5) -> (163, 366.8)
  line L120 (160.55, 366.8) -> (160.55, 365.5)
  line L121 (163, 366.8) -> (160.55, 366.8)
  line L122 (168, 365.5) -> (168, 362.5)
  line L123 (168, 545.5) -> (168, 542.5)
  line L124 (168, 365.5) -> (168, 362.5)
  point P0 (0, 0)
  point P1 (168, 364)
  dimension "d22" = 5
  dimension "d23" = 4
  dimension "d24" = 70
  dimension "d25" = 70
  dimension "d26" = 70
  dimension "d27" = 4
  dimension "d28" = 70
  dimension "d29" = 35
  dimension "d30" = 5
  dimension "d31" = 3
  dimension "d32" = 5.6
  dimension "d33" = 8.5
  dimension "d34" = 7.45
  dimension "d35" = 7.45
  dimension "d38" = 180
  dimension "d43" = 336
  dimension "d44" = 168
  constraints: 130 end point, 36 point on line, 29 symmetric about line, 8 perpendicular, 6 parallel, 4 collinear, 4 horizontal, 3 midpoint, 3 vertical, 31 other
  measures "d22" distance between parallel lines of L27 L25
  measures "d23" distance between parallel lines of L56 L58
  measures "d24" distance between parallel lines of L57 L53
  measures "d25" distance between parallel lines of L55 L59
  measures "d26" distance between parallel lines of L7 L64
  measures "d27" distance between parallel lines of L63 L8
  measures "d28" distance between parallel lines of L9 L62
  measures "d29" distance between parallel lines of L53 L68
  measures "d30" distance between parallel lines of L54 L70
  measures "d31" distance between parallel lines of L79 L69
  measures "d32" distance between parallel lines of L77 L71
  measures "d33" distance between parallel lines of L54 L74
  measures "d34" distance between parallel lines of L53 L49
  measures "d35" distance between parallel lines of L54 L72
  measures "d38" distance of L81.start L82.start
  measures "d43" distance between parallel lines of L54 L8
  measures "d44" distance between parallel lines of L54 L97
extrude "Выдавливание3" cut sketch "Эскиз5" against normal blind 4 contours L54 L90 L92 L94 L93 L91 L88 L83 L85 L86 L87 L84 | L111 L114 L113 L112 L110 L115 L118 L120 L121 L119 L117 L8 | L54 L69 L70 L71 L72 L73 L74 L75 L76 L77 L78 L79 | L109 L108 L107 L106 L105 L104 L103 L102 L101 L100 L99 L8
extrude "Выдавливание4" add sketch "Эскиз5" against normal blind 4 contours L59 L58 L57 L54 | L8 L62 L63 L64
sketch "Эскиз6" plane through (0, 0, 0) normal (0, 0, 1) x (1, 0, 0)
  line L0 (-172, 455.5) -> (-169.5, 455.5)
  line L1 (-169.5, 452.5) -> (-172, 452.5)
  line L2 (169.5, 455.5) -> (172, 455.5)
  line L3 (172, 452.5) -> (169.5, 452.5)
  line L4 (168, 454) -> (168, 454)
  arc A0 (169.5, 455.5) -> (168, 454) centre (169.5, 454) ccw
  arc A1 (168, 454) -> (169.5, 452.5) centre (169.5, 454) ccw
  line L5 (-168, 454) -> (-168, 454)
  line L6 (-172, 455.5) -> (-172, 452.5)
  line L7 (-172, 399) -> (-172, 509) projected
  arc A2 (-168, 454) -> (-169.5, 455.5) centre (-169.5, 454) ccw
  arc A3 (-169.5, 452.5) -> (-168, 454) centre (-169.5, 454) ccw
  line L8 (172, 455.5) -> (172, 452.5)
  line L9 (172, 399) -> (172, 509) projected
  point P0 (0, 0)
  dimension "d49" = 1.5
  dimension "d50" = 1.5
  constraints: 16 end point, 8 point on circle, 8 tangent, 4 centre point, 2 collinear, 2 concentric, 2 vertical
  measures "d49" radius of A0
  measures "d50" radius of A2
extrude "Выдавливание5" cut sketch "Эскиз6" against normal blind 4
